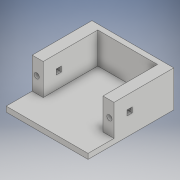
# Autodesk Inventor part: TIBIA
Saved by Autodesk Inventor 2017 (Build 210142000, 142)
## iProperties
Created: 2017-09-24
Part Number: TIBIA
Material: Generic
Document SubType Name: Modeling
Designer: Alexander Miller
Density: 1 g/cm^3
Appearance: Default
Author: Alexander Miller
Autodesk Inventor part; units mm, degrees
ref_plane "YZ Plane" through (0, 0, 0) normal (1, 0, 0) x (0, 1, 0)
ref_plane "XZ Plane" through (0, 0, 0) normal (0, 1, 0) x (-1, 0, 0)
ref_plane "XY Plane" through (0, 0, 0) normal (0, 0, 1) x (1, 0, 0)
sketch "Sketch1" plane through (0, 0, 0) normal (0, 1, 0) x (-1, 0, 0)
  line L0 (16.5, 15.75) -> (-16.5, 15.75)
  line L1 (-16.5, 15.75) -> (-16.5, -15.75)
  line L2 (-16.5, -15.75) -> (16.5, -15.75)
  line L3 (16.5, -15.75) -> (16.5, 15.75)
  point P0 (0, 0)
  point P1 (16.5, 0)
  point P2 (0, -15.75)
  dimension "d0" = 31.5
  dimension "d1" = 33
  constraints: 8 end point, 2 midpoint, 2 parallel, 1 horizontal, 1 horizontal alignment, 1 perpendicular, 1 vertical alignment
  measures "d0" distance of L0.end L1.end
  measures "d1" distance of L1.end L2.end
extrude "Extrusion1" add sketch "Sketch1" along normal blind 2
sketch "Sketch2" plane through (0, 2, 0) normal (0, 1, 0) x (1, 0, 0)
  line L0 (-6.5, 15.75) -> (14.5, 15.75)
  line L1 (14.5, 15.75) -> (14.5, 11.5)
  line L2 (14.5, 11.5) -> (-6.5, 11.5)
  line L3 (-6.5, 11.5) -> (-6.5, 15.75)
  line L4 (14.5, 15.75) -> (16.5, 15.75)
  line L5 (16.5, 15.75) -> (16.5, -15.75)
  line L6 (16.5, -15.75) -> (14.5, -15.75)
  line L7 (14.5, -15.75) -> (14.5, 15.75)
  line L8 (14.5, -11.5) -> (-6.5, -11.5)
  line L9 (-6.5, -11.5) -> (-6.5, -15.75)
  line L10 (-6.5, -15.75) -> (14.5, -15.75)
  line L11 (14.5, -15.75) -> (14.5, -11.5)
  line L12 (16.5, -15.75) -> (16.5, 15.75) projected
  line L13 (16.5, 15.75) -> (-16.5, 15.75) projected
  line L14 (-16.5, -15.75) -> (16.5, -15.75) projected
  point P0 (0, 0)
  dimension "d4" = 2
  dimension "d5" = 21
  dimension "d6" = 4.25
  constraints: 24 end point, 7 collinear, 6 parallel, 3 horizontal, 3 perpendicular, 2 equal length
  measures "d4" distance between parallel lines of L5 L7
  measures "d5" distance of L1.end L2.end
  measures "d6" distance of L2.end L0.start
extrude "Extrusion2" add sketch "Sketch2" along normal blind 12
sketch "Sketch3" plane through (-6.5, 2, -15.75) normal (-1, 0, 0) x (0, 0, 1)
  circle A0 centre (1.75, 6) radius 1
  circle A1 centre (29.75, 6) radius 1
  line L0 (4.25, 0) -> (4.25, 12) projected
  line L1 (27.25, 0) -> (27.25, 12) projected
  point P0 (15.75, -2)
  point P1 (4.25, 6)
  dimension "d9" = 2
  dimension "d10" = 1.5
  dimension "d11" = 1.5
  constraints: 2 centre point, 2 horizontal alignment, 1 equal radius, 1 midpoint
  measures "d9" diameter of A0
  measures "d10" distance edge to line of A0 L0
  measures "d11" distance edge to line of A1 L1
extrude "Extrusion3" cut sketch "Sketch3" against normal blind 10
sketch "Sketch4" plane through (-16.5, 0, 15.75) normal (0, 0, 1) x (1, 0, 0)
  line L0 (15, 9) -> (17, 9)
  line L1 (17, 9) -> (17, 7)
  line L2 (17, 7) -> (15, 7)
  line L3 (15, 7) -> (15, 9)
  line L4 (10, 2) -> (10, 14) projected
  point P0 (16.5, 0)
  point P1 (15, 8)
  point P2 (10, 8)
  dimension "d14" = 2
  dimension "d15" = 2
  dimension "d16" = 5
  constraints: 8 end point, 2 midpoint, 2 parallel, 1 horizontal, 1 horizontal alignment, 1 perpendicular
  measures "d14" distance of L0.start L0.end
  measures "d15" distance of L2.end L0.start
  measures "d16" distance between parallel lines of L4 L3
extrude "Extrusion4" cut sketch "Sketch4" against normal through all
equation "\"d0\" = servo_D"
equation "\"d1\" = servo_P"
equation "\"d5\" = servo_E"
equation "\"d6\" = -0.5 * servo_A + 0.5 * servo_D"
equation "\"d7\" = servo_B"
equation "\"d9\" = servo_H"
equation "\"d10\" = servo_L"
equation "\"d11\" = servo_L"
equation "\"servo_D\" = 31.5"
equation "\"servo_P\" = 33"
equation "\"servo_E\" = 21"
equation "\"servo_A\" = 23"
equation "\"servo_B\" = 12"
equation "\"servo_H\" = 2"
equation "\"servo_L\" = 1.5"
body "Solid1"
